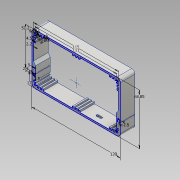
# Autodesk Inventor part: SZOMK-AK-C-C39
Saved by Autodesk Inventor 2016 (Build 200138000, 138)
## iProperties
Created: 2016-04-01
Part Number: SZOMK-AK-C-C39
Material: Aluminum 6061
Document SubType Name: Modeling
Designer: admin
Density: 2.7 g/cm^3
Appearance: Aluminum - Flat
Author: admin
Autodesk Inventor part; units mm, degrees
ref_plane "YZ Plane" through (0, 0, 0) normal (1, 0, 0) x (0, 1, 0)
ref_plane "XZ Plane" through (0, 0, 0) normal (0, 1, 0) x (-1, 0, 0)
ref_plane "XY Plane" through (0, 0, 0) normal (0, 0, 1) x (1, 0, 0)
sketch "Sketch1" plane through (0, 0, 0) normal (0, 1, 0) x (-1, 0, 0)
  arc A0 (55.5973, 28.6788) -> (54.2538, 30.0223) centre (55.5, 29.925) ccw
  arc A1 (-54.2538, 30.0223) -> (-55.5973, 28.6788) centre (-55.5, 29.925) ccw
  arc A2 (54.2538, -30.0223) -> (55.5973, -28.6788) centre (55.5, -29.925) ccw
  arc A3 (-55.5973, -28.6788) -> (-54.2538, -30.0223) centre (-55.5, -29.925) ccw
  line L0 (55.5, 34.425) -> (-55.5, 34.425)
  line L1 (55.5, -34.425) -> (-55.5, -34.425)
  line L2 (9.5866, 0) -> (-6.7847, 0) construction
  line L3 (0, -6.6233) -> (0, 6.4737) construction
  arc A4 (55.5, -34.425) -> (60, -29.925) centre (55.5, -29.925) ccw
  arc A5 (60, 29.925) -> (55.5, 34.425) centre (55.5, 29.925) ccw
  arc A6 (-55.5, 34.425) -> (-60, 29.925) centre (-55.5, 29.925) ccw
  arc A7 (-60, -29.925) -> (-55.5, -34.425) centre (-55.5, -29.925) ccw
  line L4 (57.5, 27.225) -> (57.5, 25.225)
  line L5 (57.5, 25.225) -> (55.5, 25.225)
  line L6 (55.5, 25.225) -> (55.5, 23.225)
  line L7 (55.5, 23.225) -> (57.5, 23.225)
  line L8 (57.5, 23.225) -> (57.5, 21.225)
  line L9 (57.5, 21.225) -> (55.5, 21.225)
  line L10 (55.5, 21.225) -> (55.5, 19.225)
  line L11 (55.5, 19.225) -> (57.8, 19.225)
  line L12 (57.8, 19.225) -> (57.8, -3.3607)
  line L13 (-57.5, 27.225) -> (-57.5, 25.225)
  line L14 (-57.5, 25.225) -> (-55.5, 25.225)
  line L15 (-55.5, 25.225) -> (-55.5, 23.225)
  line L16 (-55.5, 23.225) -> (-57.5, 23.225)
  line L17 (-57.5, 23.225) -> (-57.5, 21.225)
  line L18 (-57.5, 21.225) -> (-55.5, 21.225)
  line L19 (-55.5, 21.225) -> (-55.5, 19.225)
  line L20 (-55.5, 19.225) -> (-57.8, 19.225)
  line L21 (-57.8, 19.225) -> (-57.8, -3.3607)
  line L22 (57.5, 27.225) -> (55.3506, 27.225)
  line L23 (52.8, 29.7756) -> (52.8, 31.925)
  line L24 (52.8, 31.925) -> (50.8, 31.925)
  line L25 (50.8, 31.925) -> (50.8, 29.925)
  line L26 (50.8, 29.925) -> (48.8, 29.925)
  line L27 (48.8, 29.925) -> (48.8, 31.925)
  line L28 (48.8, 31.925) -> (46.8, 31.925)
  line L29 (46.8, 31.925) -> (46.8, 29.925)
  line L30 (46.8, 29.925) -> (44.8, 29.925)
  line L31 (44.8, 29.925) -> (44.8, 32.325)
  line L32 (44.8, 32.325) -> (5, 32.325)
  line L33 (5, 32.325) -> (5, 29.925)
  line L34 (5, 29.925) -> (3, 29.925)
  line L35 (3, 29.925) -> (3, 31.925)
  line L36 (3, 31.925) -> (1, 31.925)
  line L37 (1, 31.925) -> (1, 29.925)
  line L38 (1, 29.925) -> (-1, 29.925)
  line L39 (-1, 29.925) -> (-1, 31.925)
  line L40 (-1, 31.925) -> (-3, 31.925)
  line L41 (-3, 31.925) -> (-3, 29.925)
  line L42 (-3, 29.925) -> (-5, 29.925)
  line L43 (-5, 29.925) -> (-5, 32.325)
  line L44 (-5, 32.325) -> (-44.8, 32.325)
  line L45 (-44.8, 32.325) -> (-44.8, 29.925)
  line L46 (-44.8, 29.925) -> (-46.8, 29.925)
  line L47 (-46.8, 29.925) -> (-46.8, 31.925)
  line L48 (-46.8, 31.925) -> (-48.8, 31.925)
  line L49 (-48.8, 31.925) -> (-48.8, 29.925)
  line L50 (-48.8, 29.925) -> (-50.8, 29.925)
  line L51 (-50.8, 29.925) -> (-50.8, 31.925)
  line L52 (-50.8, 31.925) -> (-52.8, 31.925)
  line L53 (-52.8, 31.925) -> (-52.8, 29.7756)
  line L54 (-55.3506, 27.225) -> (-57.5, 27.225)
  line L55 (55.5973, 28.6788) -> (54.9971, 28.0786)
  line L56 (54.2538, 30.0223) -> (53.6536, 29.4221)
  line L57 (55.5, 29.925) -> (51.9091, 26.3341) construction
  arc A8 (52.8, 29.7756) -> (53.6536, 29.4221) centre (53.3, 29.7756) ccw
  arc A9 (54.9971, 28.0786) -> (55.3506, 27.225) centre (55.3506, 27.725) ccw
  line L58 (-55.5973, 28.6788) -> (-54.9971, 28.0786)
  line L59 (-54.2538, 30.0223) -> (-53.6536, 29.4221)
  arc A10 (-53.6536, 29.4221) -> (-52.8, 29.7756) centre (-53.3, 29.7756) ccw
  arc A11 (-55.3506, 27.225) -> (-54.9971, 28.0786) centre (-55.3506, 27.725) ccw
  line L60 (57.8, -3.3607) -> (55, -7.6074)
  line L61 (55, -7.6074) -> (55, -16.775)
  arc A12 (56.5, -18.525) -> (58.5, -18.525) centre (57.5, -19.275) ccw
  line L62 (58.5, -18.525) -> (58.5, -16.775)
  line L63 (56.5, -18.525) -> (56.5, -16.775)
  line L64 (55, -16.775) -> (56.5, -16.775)
  line L65 (58.5, -16.775) -> (60, -16.775)
  line L66 (57.5, -16.4962) -> (57.5, -11.7384) construction
  line L67 (-57.8, -3.3607) -> (-55, -7.6074)
  line L68 (-55, -7.6074) -> (-55, -16.775)
  arc A13 (-56.5, -15.025) -> (-58.5, -15.025) centre (-57.5, -14.275) ccw
  line L69 (-58.5, -15.025) -> (-58.5, -16.775)
  line L70 (-56.5, -15.025) -> (-56.5, -16.775)
  line L71 (-55, -16.775) -> (-56.5, -16.775)
  line L72 (-58.5, -16.775) -> (-60, -16.775)
  line L73 (-57.5, -20.9142) -> (-57.5, -16.6435) construction
  line L74 (44.8, -32.325) -> (5, -32.325)
  line L75 (5, -32.325) -> (5, -29.925)
  line L76 (5, -29.925) -> (3, -29.925)
  line L77 (3, -29.925) -> (3, -31.925)
  line L78 (3, -31.925) -> (1, -31.925)
  line L79 (1, -31.925) -> (1, -29.925)
  line L80 (1, -29.925) -> (-1, -29.925)
  line L81 (-1, -29.925) -> (-1, -31.925)
  line L82 (-1, -31.925) -> (-3, -31.925)
  line L83 (-3, -31.925) -> (-3, -29.925)
  line L84 (-3, -29.925) -> (-5, -29.925)
  line L85 (-5, -29.925) -> (-5, -32.325)
  line L86 (-5, -32.325) -> (-44.8, -32.325)
  line L87 (55, -17.425) -> (55, -25.225)
  line L88 (55, -25.225) -> (57.5, -25.225)
  line L89 (57.5, -25.225) -> (57.5, -27.225)
  line L90 (57.5, -27.225) -> (55.3506, -27.225)
  line L91 (52.8, -29.7756) -> (52.8, -31.925)
  line L92 (52.8, -31.925) -> (50.8, -31.925)
  line L93 (50.8, -31.925) -> (50.8, -29.925)
  line L94 (50.8, -29.925) -> (48.8, -29.925)
  line L95 (48.8, -29.925) -> (48.8, -31.925)
  line L96 (48.8, -31.925) -> (46.8, -31.925)
  line L97 (46.8, -31.925) -> (46.8, -29.925)
  line L98 (46.8, -29.925) -> (44.8, -29.925)
  line L99 (44.8, -29.925) -> (44.8, -32.325)
  line L100 (-44.8, -32.325) -> (-44.8, -29.925)
  line L101 (-44.8, -29.925) -> (-46.8, -29.925)
  line L102 (-46.8, -29.925) -> (-46.8, -31.925)
  line L103 (-46.8, -31.925) -> (-48.8, -31.925)
  line L104 (-48.8, -31.925) -> (-48.8, -29.925)
  line L105 (-48.8, -29.925) -> (-50.8, -29.925)
  line L106 (-50.8, -29.925) -> (-50.8, -31.925)
  line L107 (-50.8, -31.925) -> (-52.8, -31.925)
  line L108 (-52.8, -31.925) -> (-52.8, -29.7756)
  line L109 (-55.3506, -27.225) -> (-57.5, -27.225)
  line L110 (-57.5, -27.225) -> (-57.5, -25.225)
  line L111 (-57.5, -25.225) -> (-55, -25.225)
  line L112 (-55, -25.225) -> (-55, -17.425)
  line L113 (54.9971, -28.0786) -> (55.5973, -28.6788)
  line L114 (53.6536, -29.4221) -> (54.2538, -30.0223)
  arc A14 (55.3506, -27.225) -> (54.9971, -28.0786) centre (55.3506, -27.725) ccw
  arc A15 (53.6536, -29.4221) -> (52.8, -29.7756) centre (53.3, -29.7756) ccw
  line L115 (-54.2538, -30.0223) -> (-53.6536, -29.4221)
  line L116 (-55.5973, -28.6788) -> (-54.9971, -28.0786)
  arc A16 (-52.8, -29.7756) -> (-53.6536, -29.4221) centre (-53.3, -29.7756) ccw
  arc A17 (-54.9971, -28.0786) -> (-55.3506, -27.225) centre (-55.3506, -27.725) ccw
  line L117 (55, -17.425) -> (56.5, -17.425)
  line L118 (58.5, -17.425) -> (60, -17.425)
  line L119 (60, -29.925) -> (60, -17.425)
  line L120 (60, -16.775) -> (60, 29.925)
  line L121 (-55, -17.425) -> (-56.5, -17.425)
  line L122 (-56.5, -17.425) -> (-56.5, -16.775)
  line L123 (-58.5, -16.775) -> (-58.5, -17.425)
  line L124 (-58.5, -17.425) -> (-60, -17.425)
  line L125 (-60, -29.925) -> (-60, -17.425)
  line L126 (-60, -16.775) -> (-60, 29.925)
  point P0 (0, 0)
  dimension "d1" = 111
  dimension "d3" = 68.85
  dimension "d5" = 115
  dimension "d11" = 2
  dimension "d12" = 45
  dimension "d14" = 1
  dimension "d16" = 2.5
  dimension "d19" = 2.5
  dimension "d20" = 51.2
  dimension "d21" = 2
  dimension "d23" = 2.5
  dimension "d25" = 2.5
  dimension "d26" = 17
  dimension "d27" = 2.2
  dimension "d29" = 4.5
  dimension "d30" = 120
  dimension "d31" = 5
  dimension "d59" = 1.25
  dimension "d61" = 2.1
  dimension "d62" = 7.2
  dimension "d63" = 1.9
  constraints: 255 end point, 68 perpendicular, 39 collinear, 38 point on line, 36 point on circle, 34 equal length, 22 tangent, 18 centre point, 13 vertical, 11 equal radius, 11 horizontal, 9 parallel, 4 coincident, 2 horizontal alignment, 2 vertical alignment, 19 other
  measures "d1" distance of A1.centre A0.centre
  measures "d3" distance between parallel lines of L0 L1
  measures "d5" distance between parallel lines of L13 L4
  measures "d11" distance of L7.end L8.end
  measures "d12" angle of L0 L57
  measures "d14" diameter of A8
  measures "d16" distance between parallel lines of L0 L24
  measures "d19" diameter of A12
  measures "d20" distance between parallel lines of L0 L65
  measures "d21" distance between parallel lines of L62 L63
  measures "d23" distance from line of L65 A12.centre
  measures "d25" distance from line of A13.centre L72
  measures "d26" distance between parallel lines of L1 L118
  measures "d27" distance between parallel lines of L120 L12
  measures "d29" distance between parallel lines of L120 L10
  measures "d30" distance between parallel lines of L125 L119
  measures "d31" distance between parallel lines of L120 L61
  measures "d59" radius of A0
  measures "d61" distance between parallel lines of L32 L0
  measures "d62" distance between parallel lines of L22 L0
  measures "d63" distance between parallel lines of L56 L55
extrude "Extrusion1" add sketch "Sketch1" along normal blind 20 contours A0 L56 A8 L23 L24 L25 L26 L27 L28 L29 L30 L31 L32 L33 L34 L35 L36 L37 L38 L39 L40 L41 L42 L43 L44 L45 L46 L47 L48 L49 L50 L51 L52 L53 A10 L59 A1 L58 A11 L54 L13 L14 L15 L16 L17 L18 L19 L20 L21 L67 L68 L71 L70 A13 L69 L72 L126 A6 L0 A5 L120 L65 L62 A12 L63 L64 L61 L60 L12 L11 L10 L9 L8 L7 L6 L5 L4 L22 A9 L55
extrude "Extrusion2" add sketch "Sketch1" along normal blind 20 separate body contours L63 A12 L62 L118 L119 A4 L1 A7 L125 L124 L123 L69 A13 L70 L122 L121 L112 L111 L110 L109 A17 L116 A3 L115 A16 L108 L107 L106 L105 L104 L103 L102 L101 L100 L86 L85 L84 L83 L82 L81 L80 L79 L78 L77 L76 L75 L74 L99 L98 L97 L96 L95 L94 L93 L92 L91 A15 L114 A2 L113 A14 L90 L89 L88 L87 L117
sketch "Sketch2" plane through (55.5, 0, -34.425) normal (0, 0, -1) x (-1, 0, 0)
  line L0 (0, 20) -> (111, 20) projected
  line L1 (-4.5, 0) -> (-4.5, 20) projected
  line L2 (0, 0) -> (111, 0) construction
  line L3 (29.35, 9.775) -> (35.15, 9.775)
  line L4 (36, 8.925) -> (36, 7.825)
  line L5 (36, 7.825) -> (34.95, 6.775)
  line L6 (34.95, 6.775) -> (29.55, 6.775)
  line L7 (29.55, 6.775) -> (28.5, 7.825)
  line L8 (28.5, 7.825) -> (28.5, 8.925)
  arc A0 (29.35, 9.775) -> (28.5, 8.925) centre (29.35, 8.925) ccw
  arc A1 (36, 8.925) -> (35.15, 9.775) centre (35.15, 8.925) ccw
  line L9 (32.25, 33.4023) -> (32.25, 0.9977) construction
  line L10 (30.8868, 8.275) -> (33.2449, 8.275) construction
  line L11 (36.3179, 7.1) -> (28.086, 7.1) construction
  point P0 (55.5, 0)
  point P1 (28.75, 8.275)
  dimension "d49" = 7.5
  dimension "d50" = 3
  dimension "d51" = 5.4
  dimension "d52" = 45
  dimension "d53" = 1.1
  dimension "d58" = 36.75
  dimension "d65" = 0.325
  dimension "d66" = 12.9
  dimension "d67" = 11.725
  constraints: 18 end point, 4 point on circle, 4 tangent, 2 centre point, 1 equal radius, 1 horizontal, 1 point on line, 3 other
  measures "d49" distance between parallel lines of L4 L8
  measures "d50" distance between parallel lines of L6 L3
  measures "d51" distance of L5.end L6.end
  measures "d52" angle of L6 L7
  measures "d53" distance of L7.end L8.end
  measures "d58" distance between parallel lines of L1 L9
  measures "d65" distance between parallel lines of L11 L6
  measures "d66" distance between parallel lines of L0 L11
  measures "d67" distance between parallel lines of L0 L10
extrude "Extrusion3" cut sketch "Sketch2" against normal up to next bodies 2
equation "\"d16\" = d15"
equation "\"d15\" = 2.5"
body "Solid1"
body "Solid2"
